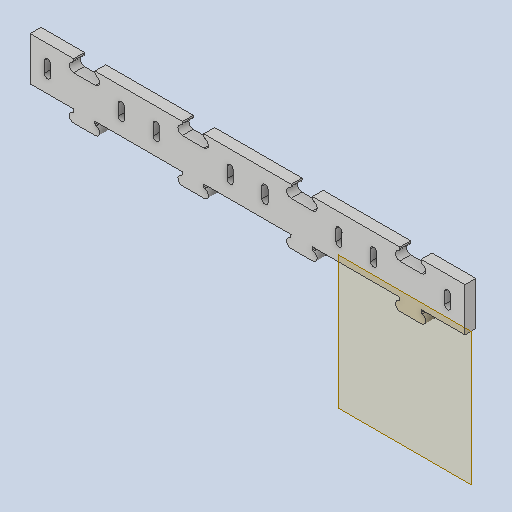
# Autodesk Inventor part: Neje_puzzle_adapterplate_v3
Saved by Autodesk Inventor 2022 (Build 260153000, 153)
## iProperties
Created: 2021-09-23
Part Number: Neje_puzzle_adapterplate_v3
Material: Generic
Document SubType Name: Modeling
Designer: diederichbenedict
Density: 1 g/cm^3
Appearance: Default
Author: diederichbenedict
Autodesk Inventor part; units mm, degrees
ref_plane "YZ Plane" through (0, 0, 0) normal (1, 0, 0) x (0, 1, 0)
ref_plane "XZ Plane" through (0, 0, 0) normal (0, 1, 0) x (-1, 0, 0)
ref_plane "XY Plane" through (0, 0, 0) normal (0, 0, 1) x (1, 0, 0)
ref_plane "Work Plane1" through (0, 0, 0) normal (0, 0, 1) x (1, 0, 0)
sketch "Sketch1" plane through (0, 0, 0) normal (0, 0, 1) x (1, 0, 0)
  circle A0 centre (-5.5948, 23.1279) radius 1.5 projected
  line L0 (30.2052, 32.2052) -> (0.2052, 32.2052) projected
  arc A1 (32.2052, 30.2052) -> (30.2052, 32.2052) centre (30.2052, 30.2052) ccw projected
  line L1 (32.2052, 30.2052) -> (32.2052, 0.2052) projected
  arc A2 (30.2052, -1.7948) -> (32.2052, 0.2052) centre (30.2052, 0.2052) ccw projected
  line L2 (15.6052, -1.7948) -> (30.2052, -1.7948) projected
  circle A3 centre (15.6052, -5.7948) radius 4 projected
  line L3 (0.2052, -1.7948) -> (15.6052, -1.7948) projected
  arc A4 (-1.7948, 0.2052) -> (0.2052, -1.7948) centre (0.2052, 0.2052) ccw projected
  line L4 (-1.7948, 0.2052) -> (-1.7948, 15.4052) projected
  circle A5 centre (-5.7948, 15.4052) radius 4 projected
  line L5 (-1.7948, 15.4052) -> (-1.7948, 30.2052) projected
  arc A6 (0.2052, 32.2052) -> (-1.7948, 30.2052) centre (0.2052, 30.2052) ccw projected
  circle A7 centre (-4.7948, -4.7948) radius 2.425 projected
  circle A8 centre (0.7052, -5.5948) radius 2.65 projected
  circle A9 centre (-5.5948, 0.7052) radius 2.65 projected
  circle A10 centre (-5.5948, 29.7052) radius 2.65 projected
  circle A11 centre (0.7052, 36.0052) radius 2.65 projected
  circle A12 centre (-4.7948, 35.2052) radius 2.425 projected
  circle A13 centre (36.0052, 0.7052) radius 2.65 projected
  circle A14 centre (29.7052, -5.5948) radius 2.65 projected
  circle A15 centre (35.2052, -4.7948) radius 2.425 projected
  circle A16 centre (36.0052, 29.7052) radius 2.65 projected
  circle A17 centre (29.7052, 36.0052) radius 2.65 projected
  circle A18 centre (35.2052, 35.2052) radius 2.425 projected
  line L6 (20.0856, 40.2052) -> (20.0856, 39.0762) projected
  arc A19 (20.0856, 39.0762) -> (20.4256, 38.6775) centre (20.4974, 39.083) ccw projected
  line L7 (20.4256, 38.6775) -> (20.5462, 38.647) projected
  arc A20 (20.0038, 34.5391) -> (20.5462, 38.647) centre (20.2052, 36.6023) ccw projected
  line L8 (20.0038, 34.5391) -> (10.2052, 34.5391) projected
  arc A21 (9.7873, 38.6768) -> (10.2052, 34.5391) centre (10.2052, 36.6291) ccw projected
  arc A22 (9.7873, 38.6768) -> (10.1151, 39.0783) centre (9.7054, 39.0783) ccw projected
  line L9 (10.1151, 39.0783) -> (10.1151, 40.2052) projected
  line L10 (10.1151, 40.2052) -> (-7.7948, 40.2052) projected
  arc A23 (-7.7948, 40.2052) -> (-9.7948, 38.2052) centre (-7.7948, 38.2052) ccw projected
  line L11 (-9.7948, 20.2052) -> (-9.7948, 38.2052) projected
  line L12 (-10.8453, 20.2052) -> (-9.7948, 20.2052) projected
  arc A24 (-11.3352, 20.6052) -> (-10.8453, 20.2052) centre (-10.8453, 20.7052) ccw projected
  arc A25 (-11.3352, 20.6052) -> (-15.2948, 20.2052) centre (-13.2948, 20.2052) ccw projected
  line L13 (-15.2948, 10.2052) -> (-15.2948, 20.2052) projected
  arc A26 (-15.2948, 10.2052) -> (-11.3352, 9.8052) centre (-13.2948, 10.2052) ccw projected
  arc A27 (-10.8453, 10.2052) -> (-11.3352, 9.8052) centre (-10.8453, 9.7052) ccw projected
  line L14 (-9.7948, 10.2052) -> (-10.8453, 10.2052) projected
  line L15 (-9.7948, -7.7948) -> (-9.7948, 10.2052) projected
  arc A28 (-9.7948, -7.7948) -> (-7.7948, -9.7948) centre (-7.7948, -7.7948) ccw projected
  line L16 (-7.7948, -9.7948) -> (10.2052, -9.7948) projected
  line L17 (10.2052, -10.8453) -> (10.2052, -9.7948) projected
  arc A29 (9.8052, -11.3352) -> (10.2052, -10.8453) centre (9.7052, -10.8453) ccw projected
  arc A30 (9.8052, -11.3352) -> (10.2052, -15.2948) centre (10.2052, -13.2948) ccw projected
  line L18 (20.2052, -15.2948) -> (10.2052, -15.2948) projected
  arc A31 (20.2052, -15.2948) -> (20.6052, -11.3352) centre (20.2052, -13.2948) ccw projected
  arc A32 (20.2052, -10.8453) -> (20.6052, -11.3352) centre (20.7052, -10.8453) ccw projected
  line L19 (20.2052, -9.7948) -> (20.2052, -10.8453) projected
  line L20 (20.2052, -9.7948) -> (38.2052, -9.7948) projected
  arc A33 (38.2052, -9.7948) -> (40.2052, -7.7948) centre (38.2052, -7.7948) ccw projected
  line L21 (40.2052, 10.3249) -> (40.2052, -7.7948) projected
  line L22 (40.2052, 10.3249) -> (39.0762, 10.3249) projected
  arc A34 (39.0762, 10.3249) -> (38.6775, 9.9849) centre (39.083, 9.9131) ccw projected
  line L23 (38.6775, 9.9849) -> (38.647, 9.8643) projected
  arc A35 (34.5391, 10.4067) -> (38.647, 9.8643) centre (36.6023, 10.2052) ccw projected
  line L24 (34.5391, 10.4067) -> (34.5391, 20.2052) projected
  arc A36 (38.6768, 20.6232) -> (34.5391, 20.2052) centre (36.6291, 20.2052) ccw projected
  arc A37 (38.6768, 20.6232) -> (39.0783, 20.2953) centre (39.0783, 20.7051) ccw projected
  line L25 (39.0783, 20.2953) -> (40.2052, 20.2953) projected
  line L26 (40.2052, 38.2052) -> (40.2052, 20.2953) projected
  arc A38 (40.2052, 38.2052) -> (38.2052, 40.2052) centre (38.2052, 38.2052) ccw projected
  line L27 (38.2052, 40.2052) -> (20.0856, 40.2052) projected
  line L28 (-149.8448, 46.2152) -> (-149.8448, 40.2152) construction
  line L29 (-149.8448, 40.2152) -> (100.1552, 40.2152) construction
  line L30 (100.1552, 46.2152) -> (100.1552, 40.2152) construction
  line L31 (-149.8448, 46.2152) -> (100.1552, 46.2152) construction
  line L32 (-149.8448, 60.2152) -> (-149.8448, 54.2152) construction
  line L33 (100.1552, 60.2152) -> (100.1552, 54.2152) construction
  line L34 (-149.8448, 60.2152) -> (100.1552, 60.2152) construction
  line L35 (-149.8448, 54.2152) -> (-149.8448, 46.2152) construction
  line L36 (-149.8448, 46.2152) -> (100.1552, 46.2152) construction
  line L37 (100.1552, 54.2152) -> (100.1552, 46.2152) construction
  line L38 (40.2052, 40.2152) -> (-9.7948, 40.2152)
  line L39 (-9.7948, 40.2152) -> (-9.7948, 60.2152)
  line L40 (-9.7948, 60.2152) -> (40.2052, 60.2152)
  line L41 (40.2052, 60.2152) -> (40.2052, 40.2152)
  circle A39 centre (15.2052, 15.2052) radius 17 construction
  line L42 (20.536, 38.598) -> (20.415, 38.6286)
  arc A40 (20.0356, 39.0758) -> (20.415, 38.6286) centre (20.4974, 39.083) ccw
  line L43 (20.0356, 39.0758) -> (20.0356, 40.2552)
  line L44 (20.0356, 40.2552) -> (38.2052, 40.2552)
  arc A41 (40.2552, 38.2052) -> (38.2052, 40.2552) centre (38.2052, 38.2052) ccw
  line L45 (40.2552, 38.2052) -> (40.2552, 20.2453)
  line L46 (40.2552, 20.2453) -> (39.0783, 20.2453)
  arc A42 (38.6278, 20.6132) -> (39.0783, 20.2453) centre (39.0783, 20.7051) ccw
  arc A43 (38.6278, 20.6132) -> (34.5891, 20.2052) centre (36.6291, 20.2052) ccw
  line L47 (34.5891, 20.2052) -> (34.5891, 10.4042)
  arc A44 (34.5891, 10.4042) -> (38.598, 9.8745) centre (36.6023, 10.2052) ccw
  line L48 (38.598, 9.8745) -> (38.6286, 9.9955)
  arc A45 (39.0758, 10.3749) -> (38.6286, 9.9955) centre (39.083, 9.9131) ccw
  line L49 (39.0758, 10.3749) -> (40.2552, 10.3749)
  line L50 (40.2552, 10.3749) -> (40.2552, -7.7948)
  arc A46 (38.2052, -9.8448) -> (40.2552, -7.7948) centre (38.2052, -7.7948) ccw
  line L51 (38.2052, -9.8448) -> (20.2552, -9.8448)
  line L52 (20.2552, -9.8448) -> (20.2552, -10.8453)
  arc A47 (20.2552, -10.8453) -> (20.6152, -11.2862) centre (20.7052, -10.8453) ccw
  arc A48 (20.2052, -15.3448) -> (20.6152, -11.2862) centre (20.2052, -13.2948) ccw
  line L53 (20.2052, -15.3448) -> (10.2052, -15.3448)
  arc A49 (9.7952, -11.2862) -> (10.2052, -15.3448) centre (10.2052, -13.2948) ccw
  arc A50 (9.7952, -11.2862) -> (10.1552, -10.8453) centre (9.7052, -10.8453) ccw
  line L54 (10.1552, -10.8453) -> (10.1552, -9.8448)
  line L55 (10.1552, -9.8448) -> (-7.7948, -9.8448)
  arc A51 (-9.8448, -7.7948) -> (-7.7948, -9.8448) centre (-7.7948, -7.7948) ccw
  line L56 (-9.8448, -7.7948) -> (-9.8448, 10.1552)
  line L57 (-9.8448, 10.1552) -> (-10.8453, 10.1552)
  arc A52 (-10.8453, 10.1552) -> (-11.2862, 9.7952) centre (-10.8453, 9.7052) ccw
  arc A53 (-15.3448, 10.2052) -> (-11.2862, 9.7952) centre (-13.2948, 10.2052) ccw
  line L58 (-15.3448, 10.2052) -> (-15.3448, 20.2052)
  arc A54 (-11.2862, 20.6152) -> (-15.3448, 20.2052) centre (-13.2948, 20.2052) ccw
  arc A55 (-11.2862, 20.6152) -> (-10.8453, 20.2552) centre (-10.8453, 20.7052) ccw
  line L59 (-10.8453, 20.2552) -> (-9.8448, 20.2552)
  line L60 (-9.8448, 20.2552) -> (-9.8448, 38.2052)
  arc A56 (-7.7948, 40.2552) -> (-9.8448, 38.2052) centre (-7.7948, 38.2052) ccw
  line L61 (-7.7948, 40.2552) -> (10.1651, 40.2552)
  line L62 (10.1651, 40.2552) -> (10.1651, 39.0783)
  arc A57 (9.7973, 38.6278) -> (10.1651, 39.0783) centre (9.7054, 39.0783) ccw
  arc A58 (9.7973, 38.6278) -> (10.2052, 34.5891) centre (10.2052, 36.6291) ccw
  line L63 (10.2052, 34.5891) -> (20.0063, 34.5891)
  arc A59 (20.0063, 34.5891) -> (20.536, 38.598) centre (20.2052, 36.6023) ccw
  line L64 (20.0356, 40.2152) -> (10.1651, 40.2152)
  point P0 (0, 0)
  dimension "d0" = 25
  dimension "d1" = 25
  dimension "d2" = 0.05
  dimension "d21" = 0
  constraints: 60 end point, 40 point on circle, 20 centre point, 4 point on line, 2 parallel, 1 collinear, 1 horizontal, 1 horizontal alignment, 1 perpendicular, 1 vertical alignment, 41 other
  measures "d0" distance from line of L39 A39.centre
  measures "d1" distance from line of A39.centre L41
  measures "d2" radial gap between concentric circles of A20 A59
  measures "d21" distance between parallel lines of L34 L40
extrude "Extrusion1" add sketch "Sketch1" against normal blind 5 contours L43 A40 L42 A59 L63 A58 A57 L62 L38 | L43 L44 A41 L38 | L38 L62 L61 A56 L39 L40 L41 A41 L44 L43 | L38 A56 L61 L62
sketch "Sketch2" plane through (0, 0, -5) normal (0, 0, -1) x (1, 0, 0)
  circle A0 centre (-5.5948, -23.1279) radius 1.5 projected
  line L0 (30.2052, -32.2052) -> (0.2052, -32.2052) construction
  arc A1 (30.2052, -32.2052) -> (32.2052, -30.2052) centre (30.2052, -30.2052) ccw projected
  line L1 (32.2052, -30.2052) -> (32.2052, -0.2052) projected
  arc A2 (32.2052, -0.2052) -> (30.2052, 1.7948) centre (30.2052, -0.2052) ccw projected
  line L2 (15.6052, 1.7948) -> (30.2052, 1.7948) projected
  circle A3 centre (15.6052, 5.7948) radius 4 projected
  line L3 (0.2052, 1.7948) -> (15.6052, 1.7948) projected
  arc A4 (0.2052, 1.7948) -> (-1.7948, -0.2052) centre (0.2052, -0.2052) ccw projected
  line L4 (-1.7948, -0.2052) -> (-1.7948, -15.4052) projected
  circle A5 centre (-5.7948, -15.4052) radius 4 projected
  line L5 (-1.7948, -15.4052) -> (-1.7948, -30.2052) projected
  arc A6 (-1.7948, -30.2052) -> (0.2052, -32.2052) centre (0.2052, -30.2052) ccw projected
  circle A7 centre (-4.7948, 4.7948) radius 2.425 projected
  circle A8 centre (0.7052, 5.5948) radius 2.65 projected
  circle A9 centre (-5.5948, -0.7052) radius 2.65 projected
  circle A10 centre (-5.5948, -29.7052) radius 2.65 projected
  circle A11 centre (0.7052, -36.0052) radius 2.65 construction
  circle A12 centre (-4.7948, -35.2052) radius 2.425 construction
  circle A13 centre (36.0052, -0.7052) radius 2.65 projected
  circle A14 centre (29.7052, 5.5948) radius 2.65 projected
  circle A15 centre (35.2052, 4.7948) radius 2.425 projected
  circle A16 centre (36.0052, -29.7052) radius 2.65 projected
  circle A17 centre (29.7052, -36.0052) radius 2.65 construction
  circle A18 centre (35.2052, -35.2052) radius 2.425 construction
  line L6 (20.0856, -40.2052) -> (20.0856, -39.0762) construction
  arc A19 (20.4256, -38.6775) -> (20.0856, -39.0762) centre (20.4974, -39.083) ccw construction
  line L7 (20.4256, -38.6775) -> (20.5462, -38.647) construction
  arc A20 (20.5462, -38.647) -> (20.0038, -34.5391) centre (20.2052, -36.6023) ccw construction
  line L8 (20.0038, -34.5391) -> (10.2052, -34.5391) construction
  arc A21 (10.2052, -34.5391) -> (9.7873, -38.6768) centre (10.2052, -36.6291) ccw construction
  arc A22 (10.1151, -39.0783) -> (9.7873, -38.6768) centre (9.7054, -39.0783) ccw construction
  line L9 (10.1151, -39.0783) -> (10.1151, -40.2052) construction
  line L10 (10.1151, -40.2052) -> (-7.7948, -40.2052) construction
  arc A23 (-9.7948, -38.2052) -> (-7.7948, -40.2052) centre (-7.7948, -38.2052) ccw construction
  line L11 (-9.7948, -20.2052) -> (-9.7948, -38.2052) projected
  line L12 (-10.8453, -20.2052) -> (-9.7948, -20.2052) projected
  arc A24 (-10.8453, -20.2052) -> (-11.3352, -20.6052) centre (-10.8453, -20.7052) ccw projected
  arc A25 (-15.2948, -20.2052) -> (-11.3352, -20.6052) centre (-13.2948, -20.2052) ccw projected
  line L13 (-15.2948, -10.2052) -> (-15.2948, -20.2052) projected
  arc A26 (-11.3352, -9.8052) -> (-15.2948, -10.2052) centre (-13.2948, -10.2052) ccw projected
  arc A27 (-11.3352, -9.8052) -> (-10.8453, -10.2052) centre (-10.8453, -9.7052) ccw projected
  line L14 (-9.7948, -10.2052) -> (-10.8453, -10.2052) projected
  line L15 (-9.7948, 7.7948) -> (-9.7948, -10.2052) projected
  arc A28 (-7.7948, 9.7948) -> (-9.7948, 7.7948) centre (-7.7948, 7.7948) ccw projected
  line L16 (-7.7948, 9.7948) -> (10.2052, 9.7948) projected
  line L17 (10.2052, 10.8453) -> (10.2052, 9.7948) projected
  arc A29 (10.2052, 10.8453) -> (9.8052, 11.3352) centre (9.7052, 10.8453) ccw projected
  arc A30 (10.2052, 15.2948) -> (9.8052, 11.3352) centre (10.2052, 13.2948) ccw projected
  line L18 (20.2052, 15.2948) -> (10.2052, 15.2948) projected
  arc A31 (20.6052, 11.3352) -> (20.2052, 15.2948) centre (20.2052, 13.2948) ccw projected
  arc A32 (20.6052, 11.3352) -> (20.2052, 10.8453) centre (20.7052, 10.8453) ccw projected
  line L19 (20.2052, 9.7948) -> (20.2052, 10.8453) projected
  line L20 (20.2052, 9.7948) -> (38.2052, 9.7948) projected
  arc A33 (40.2052, 7.7948) -> (38.2052, 9.7948) centre (38.2052, 7.7948) ccw projected
  line L21 (40.2052, -10.3249) -> (40.2052, 7.7948) projected
  line L22 (40.2052, -10.3249) -> (39.0762, -10.3249) projected
  arc A34 (38.6775, -9.9849) -> (39.0762, -10.3249) centre (39.083, -9.9131) ccw projected
  line L23 (38.6775, -9.9849) -> (38.647, -9.8643) projected
  arc A35 (38.647, -9.8643) -> (34.5391, -10.4067) centre (36.6023, -10.2052) ccw projected
  line L24 (34.5391, -10.4067) -> (34.5391, -20.2052) projected
  arc A36 (34.5391, -20.2052) -> (38.6768, -20.6232) centre (36.6291, -20.2052) ccw projected
  arc A37 (39.0783, -20.2953) -> (38.6768, -20.6232) centre (39.0783, -20.7051) ccw projected
  line L25 (39.0783, -20.2953) -> (40.2052, -20.2953) projected
  line L26 (40.2052, -38.2052) -> (40.2052, -20.2953) projected
  arc A38 (38.2052, -40.2052) -> (40.2052, -38.2052) centre (38.2052, -38.2052) ccw construction
  line L27 (38.2052, -40.2052) -> (20.0856, -40.2052) construction
  line L28 (40.2052, -40.2152) -> (20.0356, -40.2152) construction
  line L29 (10.1651, -39.0783) -> (10.1651, -40.2152) construction
  arc A39 (10.1651, -39.0783) -> (9.7973, -38.6278) centre (9.7054, -39.0783) ccw construction
  arc A40 (10.2052, -34.5891) -> (9.7973, -38.6278) centre (10.2052, -36.6291) ccw construction
  line L30 (20.0063, -34.5891) -> (10.2052, -34.5891) construction
  arc A41 (20.536, -38.598) -> (20.0063, -34.5891) centre (20.2052, -36.6023) ccw construction
  line L31 (20.415, -38.6286) -> (20.536, -38.598) construction
  arc A42 (20.415, -38.6286) -> (20.0356, -39.0758) centre (20.4974, -39.083) ccw construction
  line L32 (20.0356, -40.2152) -> (20.0356, -39.0758) construction
  line L33 (10.1651, -40.2152) -> (-9.7948, -40.2152) construction
  line L34 (40.2052, -60.2152) -> (40.2052, -40.2152) construction
  line L35 (-9.7948, -60.2152) -> (40.2052, -60.2152) construction
  line L36 (-9.7948, -40.2152) -> (-9.7948, -60.2152) construction
  line L37 (20.0356, -40.2152) -> (20.0356, -39.0758) projected
  line L38 (40.2052, -40.2152) -> (20.0356, -40.2152) projected
  line L39 (40.2052, -60.2152) -> (40.2052, -40.2152) projected
  line L40 (-9.7948, -60.2152) -> (40.2052, -60.2152) projected
  line L41 (-9.7948, -40.2152) -> (-9.7948, -60.2152) projected
  line L42 (10.1651, -40.2152) -> (-9.7948, -40.2152) projected
  line L43 (10.1651, -39.0783) -> (10.1651, -40.2152) projected
  arc A43 (10.1651, -39.0783) -> (9.7973, -38.6278) centre (9.7054, -39.0783) ccw projected
  arc A44 (10.2052, -34.5891) -> (9.7973, -38.6278) centre (10.2052, -36.6291) ccw projected
  line L44 (20.0063, -34.5891) -> (10.2052, -34.5891) projected
  arc A45 (20.536, -38.598) -> (20.0063, -34.5891) centre (20.2052, -36.6023) ccw projected
  line L45 (20.415, -38.6286) -> (20.536, -38.598) projected
  arc A46 (20.415, -38.6286) -> (20.0356, -39.0758) centre (20.4974, -39.083) ccw projected
  line L46 (-9.7948, -60.2152) -> (40.2052, -60.2152) projected
  line L47 (20.0356, -60.2152) -> (10.2651, -60.2152)
  line L48 (10.2651, -60.2152) -> (10.2651, -58.6382)
  line L49 (10.2651, -58.6382) -> (20.0356, -58.6382)
  line L50 (20.0356, -58.6382) -> (20.0356, -60.2152)
  line L51 (20.2052, -56.6152) -> (10.2052, -56.6152) construction
  line L52 (20.2052, -54.5922) -> (10.2052, -54.5922)
  line L53 (10.2052, -58.6382) -> (20.2052, -58.6382)
  arc A47 (20.2052, -58.6382) -> (20.2052, -54.5922) centre (20.2052, -56.6152) ccw
  arc A48 (10.2052, -54.5922) -> (10.2052, -58.6382) centre (10.2052, -56.6152) ccw
  line L54 (38.2052, -40.2052) -> (20.0856, -40.2052) projected
  point P0 (0, 0)
  point P1 (15.2052, -56.6152)
  dimension "d5" = 2.023
  dimension "d6" = 0
  dimension "d7" = 0
  dimension "d8" = 3.6
  dimension "d9" = 0
  dimension "d10" = 0.1
  dimension "d11" = 0
  constraints: 16 end point, 4 point on circle, 4 tangent, 3 parallel, 2 centre point, 2 horizontal, 1 horizontal alignment, 1 midpoint, 1 perpendicular, 1 point on line, 1 vertical alignment
  measures "d5" radius of A47
  measures "d6" horizontal distance of L51.start A41.centre
  measures "d7" horizontal distance of L51.end A40.centre
  measures "d8" distance from line of L35 L51.start
  measures "d9" distance between parallel lines of L50 L32
  measures "d10" distance between parallel lines of L29 L48
  measures "d11" distance between parallel lines of L53 L49
extrude "Extrusion2" cut sketch "Sketch2" against normal blind 5 contours L40 L48 L49 L50 | L49 L53 A48 L52 A47
fillet "Fillet1" radius 1 2 edges at (20.0356, 58.6382, -2.5) (10.2651, 58.6382, -2.5)
sketch "Sketch3" plane through (0, 0, -5) normal (0, 0, -1) x (-1, 0, 0)
  line L0 (149.8448, 46.2152) -> (149.8448, 54.2152) projected
  line L1 (149.8448, 54.2152) -> (-100.1552, 54.2152) projected
  line L2 (-100.1552, 46.2152) -> (-100.1552, 54.2152) projected
  line L3 (149.8448, 46.2152) -> (-100.1552, 46.2152) projected
  circle A0 centre (-32.2052, 50.2152) radius 1.45
  circle A1 centre (1.7948, 50.2152) radius 1.4
  line L4 (-40.2052, 60.2152) -> (-40.2052, 40.2152) projected
  line L5 (9.7948, 40.2152) -> (9.7948, 60.2152) projected
  ellipse E0 centre (-32.2052, 50.2152) end of major axis (-32.2052, 47.9152) minor radius 1.4189
  ellipse E1 centre (1.7948, 50.2152) end of major axis (1.7948, 52.4358) minor radius 1.4
  line L6 (1.7948, 47.6618) -> (1.7948, 52.7687) construction
  line L7 (3.2448, 47.6618) -> (3.2448, 52.7687)
  line L8 (0.3448, 52.7687) -> (0.3448, 47.6618)
  arc A2 (0.3448, 47.6618) -> (3.2448, 47.6618) centre (1.7948, 47.6618) ccw
  arc A3 (3.2448, 52.7687) -> (0.3448, 52.7687) centre (1.7948, 52.7687) ccw
  line L9 (-32.2052, 47.6618) -> (-32.2052, 52.7687) construction
  line L10 (-33.6242, 47.6618) -> (-33.6242, 52.7687)
  line L11 (-30.7863, 52.7687) -> (-30.7863, 47.6618)
  arc A4 (-33.6242, 47.6618) -> (-30.7863, 47.6618) centre (-32.2052, 47.6618) ccw
  arc A5 (-30.7863, 52.7687) -> (-33.6242, 52.7687) centre (-32.2052, 52.7687) ccw
  point P0 (0, 0)
  dimension "d25" = 2.3
  dimension "d15" = 2.9
  dimension "d16" = 2.8
  dimension "d17" = 8
  dimension "d18" = 8
  dimension "d26" = 2.9
  constraints: 16 end point, 8 point on circle, 8 tangent, 6 centre point, 3 vertical, 2 coincident, 2 midpoint, 2 parallel, 5 other
  measures "d15" diameter of A0
  measures "d16" diameter of A1
  measures "d17" distance from line of A0.centre L4
  measures "d18" distance from line of L5 A1.centre
  measures "d26" diameter of A3
extrude "Extrusion3" cut sketch "Sketch3" against normal through all contours A2 L3 | L3 A2 L8 A3 L1 L7 | L1 A3 | L11 E0 A0 | A0 E0 L10 A5 L11 | L11 A4 L10 A0 E0 | A0 E0 L11 | E0 A0 | A0 E0 | E0 A0 | E0 L10 A0 | A0 L10 E0 | A1 | E1 A1 | A1 E1
pattern_linear "Rectangular Pattern1" count 4 spacing 50 along (-1, 0, 0) of "Extrusion2", "Fillet1", "Extrusion3", "Extrusion1"
body "Solid1"
